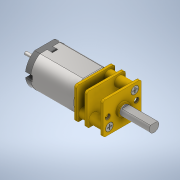
# Autodesk Inventor part: Pololu_MicroMotor
Saved by Autodesk Inventor 2020 (Build 240168000, 168)
## iProperties
Created: 2020-01-30
Part Number: Pololu_MicroMotor
Material: Generic
Document SubType Name: Modeling
Designer: ermoz
Density: 1 g/cm^3
Appearance: Default
Mass: 2.06748 g
Surface Area: 20.9701 cm^2
Volume: 2.06748 cm^3
Author: ermoz
Autodesk Inventor part; units mm, degrees
ref_plane "YZ Plane" through (0, 0, 0) normal (1, 0, 0) x (0, 1, 0)
ref_plane "XZ Plane" through (0, 0, 0) normal (0, 1, 0) x (-1, 0, 0)
ref_plane "XY Plane" through (0, 0, 0) normal (0, 0, 1) x (1, 0, 0)
sketch "Sketch1" plane through (0, 0, 0) normal (1, 0, 0) x (0, 1, 0)
  circle A0 centre (0, 0) radius 6
  line L0 (5.1371, 3.1) -> (5.1371, -3.1)
  line L1 (-5.1371, -3.1) -> (-5.1371, 3.1)
  line L2 (-5.1371, 3.1) -> (5.1371, -3.1) construction
  line L3 (5.1371, 3.1) -> (-5.1371, -3.1) construction
  constraints: 8 end point, 2 midpoint, 1 coincident, 1 parallel, 3 other
extrude "Extrusion1" add sketch "Sketch1" along normal blind 15.4 contours L0 A0 L1
fillet "Fillet1" radius 0.2 4 edges at (15.4, 0, 6) (15.4, 0, -6) (15.4, 5.1371, 0) (15.4, -5.1371, 0)
sketch "Sketch2" plane through (15.4, 0, 0) normal (1, 0, 0) x (0, 0, -1)
  line L0 (-6, -5) -> (6, -5)
  line L1 (6, -5) -> (6, 5)
  line L2 (6, 5) -> (-6, 5)
  line L3 (-6, 5) -> (-6, -5)
  line L4 (-6, -5) -> (6, 5) construction
  line L5 (6, -5) -> (-6, 5) construction
  point P0 (0, 0)
  dimension "d5" = 12
  dimension "d6" = 10
  constraints: 12 end point, 2 midpoint, 2 parallel, 1 horizontal, 1 perpendicular
  measures "d5" distance of L2.end L1.end
  measures "d6" distance of L1.end L0.end
extrude "Extrusion2" add sketch "Sketch2" along normal blind 0.75 separate body
sketch "Sketch3" plane through (16.15, 0, 0) normal (1, 0, 0) x (0, 0, -1)
  line L0 (6, -5) -> (6, 5) projected
  line L1 (-6, -5) -> (6, -5)
  line L2 (6, -5) -> (6, 5)
  line L3 (6, 5) -> (-6, 5)
  line L4 (-6, 5) -> (-6, -5)
  line L5 (-6, -5) -> (6, 5) construction
  line L6 (6, -5) -> (-6, 5) construction
  point P0 (0, 0)
  constraints: 12 end point, 2 midpoint, 2 parallel, 1 horizontal, 1 perpendicular
extrude "Extrusion3" add sketch "Sketch3" along normal blind 8.25 bodies 2
sketch "Sketch4" plane through (15.4, 5, 6) normal (0, 1, 0) x (1, 0, 0)
  line L0 (0, 12) -> (9, 12) projected
  line L1 (0, 0) -> (0.75, 0)
  line L2 (0.75, 0) -> (0.75, 12)
  line L3 (0.75, 12) -> (0, 12)
  line L4 (0, 12) -> (0, 0)
  line L5 (9, 0) -> (9, 12) projected
  line L6 (9, 0) -> (8.25, 0)
  line L7 (8.25, 0) -> (8.25, 12)
  line L8 (8.25, 12) -> (9, 12)
  line L9 (9, 12) -> (9, 0)
  line L10 (4.875, 12) -> (4.125, 12)
  line L11 (4.125, 12) -> (4.125, 0)
  line L12 (4.125, 0) -> (4.875, 0)
  line L13 (4.875, 0) -> (4.875, 12)
  line L14 (4.875, 12) -> (4.125, 0) construction
  line L15 (4.125, 12) -> (4.875, 0) construction
  line L16 (8.25, 0) -> (4.875, 0)
  line L17 (4.875, 0) -> (4.875, 12)
  line L18 (4.875, 12) -> (8.25, 12)
  line L19 (8.25, 12) -> (8.25, 0)
  line L20 (4.125, 0) -> (0.75, 0)
  line L21 (0.75, 0) -> (0.75, 12)
  line L22 (0.75, 12) -> (4.125, 12)
  line L23 (4.125, 12) -> (4.125, 0)
  point P0 (-15.4, 6)
  point P1 (4.5, 6)
  point P2 (0.75, 0)
  point P3 (4.125, 12)
  point P4 (4.875, 0)
  point P5 (8.25, 12)
  point P6 (4.875, 12)
  dimension "d11" = 0.75
  dimension "d12" = 0.75
  dimension "d13" = 0.75
  constraints: 44 end point, 10 parallel, 5 horizontal, 5 perpendicular, 2 midpoint, 2 point on line
  measures "d11" distance of L3.end L2.end
  measures "d12" distance of L7.end L8.end
  measures "d13" distance of L12.end L11.end
extrude "Extrusion4" cut sketch "Sketch4" against normal blind 10 contours L0 L11 L20 L2 | L0 L7 L16 L13 bodies 2
sketch "Sketch5" plane through (24.4, 0, 0) normal (1, 0, 0) x (0, 0, -1)
  line L0 (6, -5) -> (6, 5) projected
  line L1 (6, 5) -> (4, 5)
  line L2 (4, 5) -> (4, 3)
  line L3 (4, 3) -> (6, 3)
  line L4 (6, 3) -> (6, 5)
  circle A0 centre (4, 3) radius 1.5
  line L5 (-6, 5) -> (-6, -5) projected
  line L6 (-6, -5) -> (-4, -5)
  line L7 (-4, -5) -> (-4, -3)
  line L8 (-4, -3) -> (-6, -3)
  line L9 (-6, -3) -> (-6, -5)
  circle A1 centre (-4, -3) radius 1.5
  point P0 (0, 0)
  dimension "d16" = 2
  dimension "d17" = 2
  dimension "d18" = 3
  dimension "d19" = 2
  dimension "d20" = 2
  dimension "d21" = 3
  constraints: 16 end point, 4 parallel, 2 centre point, 2 coincident, 2 horizontal, 2 perpendicular
  measures "d16" distance of L3.end L2.end
  measures "d17" distance of L2.end L1.end
  measures "d18" diameter of A0
  measures "d19" distance of L8.end L7.end
  measures "d20" distance of L7.end L6.end
  measures "d21" diameter of A1
extrude "Extrusion5" add sketch "Sketch5" against normal blind 9 contours A0 L2 L3 | L3 L2 A0 | A1 L7 L8 | L8 L7 A1 bodies 2
fillet "Fillet2" radius 0.75 12 edges at (24.025, 5, -6) (19.9, 5, -6) (15.775, 5, -6) (24.025, -5, -6) (19.9, -5, -6) (15.775, -5, -6) (24.025, -5, 6) (19.9, -5, 6) (15.775, -5, 6) (19.9, 5, 6) (15.775, 5, 6) (24.025, 5, 6)
sketch "Sketch6" plane through (24.4, 0, 0) normal (1, 0, 0) x (0, 0, -1)
  circle A0 centre (0, 0) radius 2
  circle A1 centre (0, 0) radius 1.5
  dimension "d25" = 4
  dimension "d26" = 3
  constraints: 2 centre point, 2 coincident
  measures "d25" diameter of A0
  measures "d26" diameter of A1
extrude "Extrusion6" add sketch "Sketch6" along normal blind 0.7 bodies 2
extrude "Extrusion7" add sketch "Sketch6" along normal blind 10 separate body contours A1
sketch "Sketch7" plane through (34.4, 0, 0) normal (1, 0, 0) x (0, 0, -1)
  line L0 (-2.6164, 2) -> (2.6164, 2)
  line L1 (2.6164, 2) -> (2.6164, 1)
  line L2 (2.6164, 1) -> (-2.6164, 1)
  line L3 (-2.6164, 1) -> (-2.6164, 2)
  circle A0 centre (0, 0) radius 1.5 projected
  line L4 (-2.6164, 2) -> (2.6164, 1) construction
  line L5 (2.6164, 2) -> (-2.6164, 1) construction
  point P0 (0, 1.5)
  point P1 (-1.118, 1)
  point P2 (1.118, 1)
  dimension "d31" = 1
  constraints: 12 end point, 2 midpoint, 2 parallel, 1 horizontal, 1 perpendicular, 2 other
  measures "d31" distance of L0.end L1.end
extrude "Extrusion8" cut sketch "Sketch7" against normal blind 9 contours A0 L2 picked at (-0.2826, 1.0791) bodies 3
sketch "Sketch8" plane through (24.4, 0, 0) normal (1, 0, 0) x (0, 0, -1)
  circle A0 centre (-4.5, 0) radius 0.8
  circle A1 centre (4.5, 0) radius 0.8
  point P0 (0, 0)
  dimension "d35" = 1.6
  dimension "d36" = 1.6
  constraints: 2 centre point
  measures "d35" diameter of A0
  measures "d36" diameter of A1
extrude "Extrusion9" cut sketch "Sketch8" against normal blind 1 bodies 2
thread "Thread1" size "M1.6x0.35" class "6H" standard "ANSI Metric M Profile" full length
thread "Thread2" size "M1.6x0.35" class "6H" standard "ANSI Metric M Profile" full length
sketch "Sketch9" plane through (24.4, 0, 0) normal (1, 0, 0) x (0, 0, -1)
  circle A0 centre (4, 3) radius 1.5 projected
  circle A1 centre (4, 3) radius 0.5
  circle A2 centre (-4, -3) radius 1.5 projected
  circle A3 centre (-4, -3) radius 0.5
  point P0 (0, 0)
  dimension "d43" = 1
  dimension "d44" = 1
  constraints: 2 centre point, 2 coincident
  measures "d43" diameter of A1
  measures "d44" diameter of A3
extrude "Extrusion10" cut sketch "Sketch9" against normal blind 1.5 contours A1 | A3 bodies 2
chamfer "Chamfer1" distance 0.75 angle 45 2 edges at (24.4, 3, -3.5) (24.4, -3, 4.5)
sketch "Sketch10" plane through (22.9, 3, -4) normal (1, 0, 0) x (0, 0, -1)
  circle A0 centre (0, 0) radius 0.5
  circle A1 centre (-8, -6) radius 0.5 projected
  circle A2 centre (-8, -6) radius 0.5
  point P0 (-4, -3)
  constraints: 2 centre point, 1 coincident
extrude "Extrusion11" add sketch "Sketch10" along normal blind 1.5 separate body
sketch "Sketch11" plane through (24.4, 3, -4) normal (1, 0, 0) x (0, 0, -1)
  circle A0 centre (0, 0) radius 1.25
  circle A1 centre (-8, -6) radius 0.5 projected
  circle A2 centre (-8, -6) radius 1.25
  point P0 (-4, -3)
  dimension "d52" = 2.5
  dimension "d53" = 2.5
  constraints: 2 centre point, 1 coincident
  measures "d52" diameter of A0
  measures "d53" diameter of A2
extrude "Extrusion12" add sketch "Sketch11" along normal blind 1 contours A0 | A1 | A2 bodies 4
chamfer "Chamfer2" distance 0.75 angle 45 2 edges at (24.4, 3, -3.5) (24.4, -3, 4.5)
sketch "Sketch12" plane through (25.4, -3, 4) normal (1, 0, 0) x (0, 0, -1)
  circle A0 centre (0, 0) radius 1.25 projected
  circle A1 centre (0, 0) radius 1.25
  circle A2 centre (8, 6) radius 1.25 projected
  circle A3 centre (8, 6) radius 1.25
  point P0 (4, 3)
  constraints: 2 centre point, 2 coincident
extrude "Extrusion13" cut sketch "Sketch12" against normal blind 1 bodies 4
fillet "Fillet3" radius 0.05 4 edges at (24.4, 3, -2.75) (24.4, -3, 5.25) (24.4, 3, -2.7505) (24.4, -3, 5.2495)
sketch "Sketch13" plane through (24.4, 3, -4) normal (1, 0, 0) x (0, 0, -1)
  line L0 (-0.75, -0.125) -> (0.75, -0.125)
  line L1 (0.75, -0.125) -> (0.75, 0.125)
  line L2 (0.75, 0.125) -> (-0.75, 0.125)
  line L3 (-0.75, 0.125) -> (-0.75, -0.125)
  circle A0 centre (0, 0) radius 0.5 projected
  line L4 (-0.75, -0.125) -> (0.75, 0.125) construction
  line L5 (0.75, -0.125) -> (-0.75, 0.125) construction
  line L6 (-0.125, -0.75) -> (0.125, -0.75)
  line L7 (0.125, -0.75) -> (0.125, 0.75)
  line L8 (0.125, 0.75) -> (-0.125, 0.75)
  line L9 (-0.125, 0.75) -> (-0.125, -0.75)
  line L10 (-0.125, -0.75) -> (0.125, 0.75) construction
  line L11 (0.125, -0.75) -> (-0.125, 0.75) construction
  line L12 (-8.75, -6.125) -> (-7.25, -6.125)
  line L13 (-7.25, -6.125) -> (-7.25, -5.875)
  line L14 (-7.25, -5.875) -> (-8.75, -5.875)
  line L15 (-8.75, -5.875) -> (-8.75, -6.125)
  circle A1 centre (-8, -6) radius 0.5 projected
  line L16 (-8.75, -6.125) -> (-7.25, -5.875) construction
  line L17 (-7.25, -6.125) -> (-8.75, -5.875) construction
  line L18 (-8.125, -6.75) -> (-7.875, -6.75)
  line L19 (-7.875, -6.75) -> (-7.875, -5.25)
  line L20 (-7.875, -5.25) -> (-8.125, -5.25)
  line L21 (-8.125, -5.25) -> (-8.125, -6.75)
  line L22 (-8.125, -6.75) -> (-7.875, -5.25) construction
  line L23 (-7.875, -6.75) -> (-8.125, -5.25) construction
  point P0 (-4, -3)
  point P1 (-0.125, -0.125)
  point P2 (0.125, -0.125)
  point P3 (0.125, 0.125)
  point P4 (-0.125, 0.125)
  point P5 (-8.125, -5.875)
  point P6 (-8.125, -6.125)
  point P7 (-7.875, -6.125)
  point P8 (-7.875, -5.875)
  dimension "d62" = 1.5
  dimension "d63" = 0.25
  dimension "d64" = 0.25
  dimension "d65" = 1.5
  dimension "d66" = 1.5
  dimension "d67" = 0.25
  dimension "d68" = 0.25
  dimension "d69" = 1.5
  constraints: 48 end point, 8 midpoint, 8 parallel, 4 horizontal, 4 perpendicular
  measures "d62" distance of L2.end L1.end
  measures "d63" distance of L1.end L0.end
  measures "d64" distance of L8.end L7.end
  measures "d65" distance of L7.end L6.end
  measures "d66" distance of L14.end L13.end
  measures "d67" distance of L13.end L12.end
  measures "d68" distance of L20.end L19.end
  measures "d69" distance of L19.end L18.end
extrude "Extrusion14" cut sketch "Sketch13" against normal blind 0.5 contours L3 L2 A0 L0 | A0 L2 L9 L0 | L9 L2 L7 L0 | L0 L7 A0 L9 | A0 L7 L6 L9 | L7 L2 A0 L0 | L9 A0 L7 L2 | L9 L8 L7 A0 | A0 L2 L1 L0 | L15 L14 A1 L12 | A1 L14 L21 L12 | L21 L14 L19 L12 | L12 L19 A1 L21 | A1 L19 L18 L21 | L19 L14 A1 L12 | L21 A1 L19 L14 | L21 L20 L19 A1 | A1 L14 L13 L12 bodies 4
sketch "Sketch14" plane through (0, 0, 0) normal (-1, 0, 0) x (0, 0, 1)
  circle A0 centre (0, 0) radius 6
  line L0 (-3.1, 5.1371) -> (3.1, 5.1371) projected
  line L1 (-3.1, 5.1371) -> (3.1, 5.1371)
  line L2 (3.1, -5.1371) -> (-3.1, -5.1371) projected
  line L3 (-3.1, -5.1371) -> (3.1, -5.1371)
  constraints: 4 end point, 2 collinear, 1 centre point, 1 coincident
extrude "Extrusion15" cut sketch "Sketch14" against normal blind 1.7 contours A0 L2 L0 bodies 1
extrude "Extrusion16" add sketch "Sketch14" against normal blind 1.7 separate body contours A0 L2 L0
sketch "Sketch15" plane through (0, 0, 0) normal (-1, 0, 0) x (0, 0, 1)
  arc A0 (1.118, 1) -> (-1.118, 1) centre (0, 0) ccw projected
  circle A1 centre (0, 0) radius 2.5
  dimension "d76" = 5
  constraints: 1 centre point, 1 coincident
  measures "d76" diameter of A1
extrude "Extrusion17" add sketch "Sketch15" along normal blind 0.8 bodies 5
sketch "Sketch16" plane through (-0.8, 0, 0) normal (-1, 0, 0) x (0, 0, 1)
  circle A0 centre (0, 0) radius 0.5
  dimension "d79" = 1
  constraints: 1 centre point, 1 coincident
  measures "d79" diameter of A0
extrude "Extrusion18" add sketch "Sketch16" along normal blind 5 separate body
sketch "Sketch17" plane through (0, 0, 0) normal (-1, 0, 0) x (0, 0, 1)
  line L0 (-3.1, 5.1371) -> (3.1, 5.1371) projected
  line L1 (-3.1, 5.1371) -> (3.1, 5.1371)
  line L2 (3.1, 5.1371) -> (3.1, -1.5)
  line L3 (3.1, -1.5) -> (-3.1, -1.5)
  line L4 (-3.1, -1.5) -> (-3.1, 5.1371)
  line L5 (-2.9, -1) -> (-3.3, -1)
  line L6 (-3.3, -1) -> (-3.3, 1)
  line L7 (-3.3, 1) -> (-2.9, 1)
  line L8 (-2.9, 1) -> (-2.9, -1)
  line L9 (-2.9, -1) -> (-3.3, 1) construction
  line L10 (-3.3, -1) -> (-2.9, 1) construction
  line L11 (3.3, -1) -> (2.9, -1)
  line L12 (2.9, -1) -> (2.9, 1)
  line L13 (2.9, 1) -> (3.3, 1)
  line L14 (3.3, 1) -> (3.3, -1)
  line L15 (3.3, -1) -> (2.9, 1) construction
  line L16 (2.9, -1) -> (3.3, 1) construction
  line L17 (-3.1, 1) -> (-3.1, -1)
  line L18 (3.1, 1) -> (3.1, -1)
  point P0 (0, 0)
  point P1 (-3.1, 0)
  point P2 (3.1, 0)
  dimension "d82" = 6.2
  dimension "d83" = 0.4
  dimension "d84" = 2
  dimension "d85" = 0.4
  dimension "d86" = 2
  constraints: 36 end point, 8 midpoint, 6 parallel, 3 horizontal, 3 perpendicular, 2 point on line
  measures "d82" distance of L2.end L3.end
  measures "d83" distance of L6.end L7.end
  measures "d84" distance of L5.end L6.end
  measures "d85" distance of L12.end L13.end
  measures "d86" distance of L11.end L12.end
extrude "Extrusion19" add sketch "Sketch17" along normal blind 1.8 separate body contours L7 L8 L5 L4 | L2 L11 L12 L13
sketch "Sketch18" plane through (0, -1, -3.1) normal (0, 0, -1) x (-1, 0, 0)
  line L0 (0, 2) -> (1.8, 2) projected
  line L1 (1.8, 2) -> (1.8, 0) projected
  line L2 (0, 2) -> (1.8, 2)
  line L3 (1.8, 2) -> (1.8, 0)
  line L4 (1.8, 0) -> (0, 0)
  line L5 (0, 0) -> (0, 2)
  circle A0 centre (0.8, 1) radius 1
  circle A1 centre (0.8, 1) radius 0.5
  point P0 (0, 1)
  point P1 (1.8, 1)
  point P2 (0.8, 0)
  point P3 (0.8, 2)
  dimension "d89" = 1
  constraints: 8 end point, 3 tangent, 2 centre point, 2 parallel, 1 coincident, 1 horizontal, 1 perpendicular
  measures "d89" diameter of A1
extrude "Extrusion20" cut sketch "Sketch18" against normal blind 10 contours L0 L1 A0 | L1 L4 A0 | A1 bodies 7
sketch "Sketch19" plane through (15.2, 5.1371, 3.1) normal (0, 1, 0) x (1, 0, 0)
  line L0 (-13.5, 6.2) -> (-13.5, 0) projected
  line L1 (-11.8, 3.95) -> (-13.5, 3.95)
  line L2 (-13.5, 3.95) -> (-13.5, 2.25)
  line L3 (-13.5, 2.25) -> (-11.8, 2.25)
  line L4 (-11.8, 2.25) -> (-11.8, 3.95)
  line L5 (-11.8, 3.95) -> (-13.5, 2.25) construction
  line L6 (-13.5, 3.95) -> (-11.8, 2.25) construction
  point P0 (-15.2, 3.1)
  point P1 (-12.65, 3.1)
  dimension "d93" = 1.7
  constraints: 12 end point, 2 midpoint, 2 parallel, 1 horizontal, 1 perpendicular, 1 point on line
  measures "d93" distance of L2.end L1.end
extrude "Extrusion21" cut sketch "Sketch19" against normal blind 0.5 bodies 1
sketch "Sketch20" plane through (0, 5.1371, 3.1) normal (0, 1, 0) x (1, 0, 0)
  line L0 (1.7, 0) -> (1.7, 6.2) projected
  line L1 (3.4, 2.25) -> (1.7, 2.25) projected
  line L2 (1.7, 3.9504) -> (3, 3.9504)
  line L3 (3, 3.9504) -> (3, 2.25)
  line L4 (3, 2.25) -> (1.7, 2.25)
  line L5 (1.7, 2.25) -> (1.7, 3.9504)
  point P0 (0, 3.1)
  dimension "d96" = 1.3
  constraints: 8 end point, 2 parallel, 2 point on line, 1 horizontal, 1 perpendicular
  measures "d96" distance of L3.end L4.end
extrude "Extrusion22" add sketch "Sketch20" against normal blind 0.5 bodies 5
sketch "Sketch21" plane through (15.2, -5.1371, -3.1) normal (0, -1, 0) x (1, 0, 0)
  line L0 (-13.5, 3.95) -> (-13.5, 2.25) projected
  line L1 (-11.8, 3.95) -> (-13.5, 3.95) projected
  line L2 (-13.5, 2.25) -> (-11.8, 2.25)
  line L3 (-11.8, 2.25) -> (-11.8, 3.95)
  line L4 (-11.8, 3.95) -> (-13.5, 3.95)
  line L5 (-13.5, 3.95) -> (-13.5, 2.25)
  point P0 (-15.2, 3.1)
  constraints: 8 end point, 2 parallel, 1 horizontal, 1 perpendicular
extrude "Extrusion23" cut sketch "Sketch21" against normal blind 0.5 bodies 1
sketch "Sketch22" plane through (0, -5.1371, -3.1) normal (0, -1, 0) x (1, 0, 0)
  line L0 (3, 3.95) -> (1.7, 3.95) projected
  line L1 (1.7, 2.2496) -> (3, 2.2496)
  line L2 (3, 2.2496) -> (3, 3.95)
  line L3 (3, 3.95) -> (1.7, 3.95)
  line L4 (1.7, 3.95) -> (1.7, 2.2496)
  point P0 (0, 3.1)
  constraints: 8 end point, 2 parallel, 1 horizontal, 1 perpendicular
extrude "Extrusion24" add sketch "Sketch22" against normal blind 0.5 bodies 5
sketch "Sketch23" plane through (0, 0, 0) normal (-1, 0, 0) x (0, 0, 1)
  line L0 (-6, -4.25) -> (-6, 4.25) projected
  circle A0 centre (-4.5, 0) radius 0.8 projected
  line L1 (-6, 0) -> (-4.5, 0)
  line L2 (-6, 0) -> (-4.5, 0)
  line L3 (-4.5, 0) -> (-4.5, 0.8)
  line L4 (-4.5, 0.8) -> (-6, 0.8)
  line L5 (-6, 0.8) -> (-6, 0)
  line L6 (-6, 0) -> (-4.5, 0)
  line L7 (-4.5, 0) -> (-4.5, -0.8)
  line L8 (-4.5, -0.8) -> (-6, -0.8)
  line L9 (-6, -0.8) -> (-6, 0)
  line L10 (6, 4.25) -> (6, -4.25) projected
  circle A1 centre (4.5, 0) radius 0.8 projected
  line L11 (6, 0) -> (4.5, 0)
  line L12 (4.5, 0) -> (4.5, 0.8)
  line L13 (4.5, 0.8) -> (6, 0.8)
  line L14 (6, 0.8) -> (6, 0)
  line L15 (6, 0) -> (4.5, 0)
  line L16 (4.5, 0) -> (4.5, -0.8)
  line L17 (4.5, -0.8) -> (6, -0.8)
  line L18 (6, -0.8) -> (6, 0)
  point P0 (0, 0)
  dimension "d103" = 1.5
  constraints: 34 end point, 8 parallel, 5 horizontal, 4 perpendicular, 2 midpoint, 2 point on circle, 2 point on line, 1 vertical alignment, 1 other
  measures "d103" distance of L1.start L1.end
extrude "Extrusion25" cut sketch "Sketch23" against normal blind 2 contours L0 L1 A0 L8 | L0 L4 A0 L1 | A0 L1 L7 | A0 L3 L1 | L10 L11 A1 L13 | L10 L17 A1 L11 | A1 L11 L12 | A1 L16 L11 bodies 5
sketch "Sketch24" plane through (1.7, 0, 0) normal (-1, 0, 0) x (0, 0, 1)
  circle A0 centre (-4.5, 0) radius 0.8 projected
  line L0 (-4.5, 0.8) -> (-6.3778, 0.8)
  line L1 (-6.3778, 0.8) -> (-6.3778, -0.8)
  line L2 (-6.3778, -0.8) -> (-4.5, -0.8)
  line L3 (-4.5, -0.8) -> (-4.5, 0.8)
  circle A1 centre (4.5, 0) radius 0.8 projected
  line L4 (4.5, 0.8) -> (7.4703, 0.8)
  line L5 (7.4703, 0.8) -> (7.4703, -0.8)
  line L6 (7.4703, -0.8) -> (4.5, -0.8)
  line L7 (4.5, -0.8) -> (4.5, 0.8)
  point P0 (0, 0)
  dimension "d106" = 1.6
  constraints: 16 end point, 4 parallel, 2 horizontal, 2 perpendicular, 2 point on line, 2 vertical alignment, 2 other
  measures "d106" distance of L1.end L0.end
extrude "Extrusion26" cut sketch "Sketch24" against normal blind 0.5 contours L3 A0 | A0 L2 L1 L0 | A1 L7 | A1 L4 L5 L6 picked at (-4.9371, -0.0718) picked at (4.6663, 0.2085) bodies 1
sketch "Sketch25" plane through (20.275, 5, 5.25) normal (1, 0, 0) x (0, 0, -1)
  circle A0 centre (1.25, -8) radius 1.5 projected
  circle A1 centre (1.25, -8) radius 1.5
  circle A2 centre (9.25, -2) radius 1.5 projected
  circle A3 centre (9.25, -2) radius 1.5
  line L0 (11.25, -10) -> (-0.75, -10)
  line L1 (-0.75, -10) -> (-0.75, 0)
  line L2 (-0.75, 0) -> (11.25, 0)
  line L3 (11.25, 0) -> (11.25, -10)
  line L4 (11.25, -10) -> (-0.75, 0) construction
  line L5 (-0.75, -10) -> (11.25, 0) construction
  point P0 (5.25, -5)
  dimension "d109" = 12
  dimension "d110" = 10
  constraints: 12 end point, 2 centre point, 2 coincident, 2 midpoint, 2 parallel, 1 horizontal, 1 perpendicular
  measures "d109" distance of L1.end L2.end
  measures "d110" distance of L0.end L1.end
extrude "Extrusion27" add sketch "Sketch25" against normal blind 1.625 bodies 2
sketch "Sketch26" plane through (20.275, 5, 6) normal (1, 0, 0) x (0, 0, -1)
  circle A0 centre (10, -2) radius 1.5 projected
  circle A1 centre (10, -2) radius 1.5
  circle A2 centre (2, -8) radius 1.5 projected
  circle A3 centre (2, -8) radius 1.5
  line L0 (0, 0) -> (12, 0) projected
  line L1 (0, -10) -> (12, -10)
  line L2 (12, -10) -> (12, 0)
  line L3 (12, 0) -> (0, 0)
  line L4 (0, 0) -> (0, -10)
  circle A4 centre (6, -5) radius 0.5 projected
  line L5 (0, -10) -> (12, 0) construction
  line L6 (12, -10) -> (0, 0) construction
  constraints: 12 end point, 2 centre point, 2 coincident, 2 midpoint, 2 parallel, 1 horizontal, 1 perpendicular
extrude "Extrusion28" cut sketch "Sketch26" against normal blind 0.875 contours L0 L2 L1 L4 | A4 bodies 2
fillet "Fillet4" radius 0.75 4 edges at (19.025, 5, 6) (19.025, 5, -6) (19.025, -5, -6) (19.025, -5, 6)
body "Solid1"
body "Solid2"
body "Solid3"
body "Solid4"
body "Solid5"
body "Solid6"
body "Solid7"
